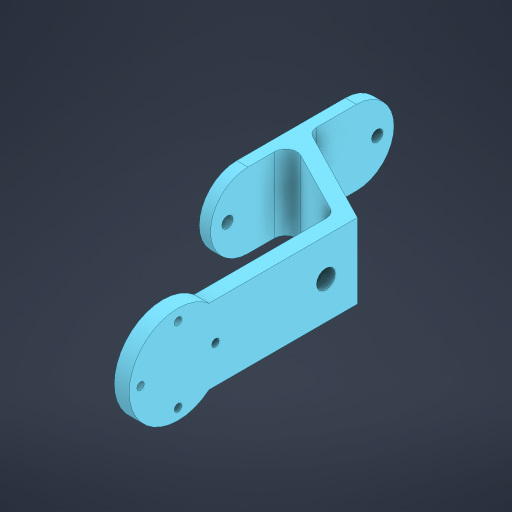
# Autodesk Inventor part: acople_3
Saved by Autodesk Inventor 2023.1 (Build 271208000, 208)
## iProperties
Created: 2022-10-29
Part Number: acople_3
Material: Generic
Document SubType Name: Modeling
Designer: amtat
Density: 1 g/cm^3
Appearance: Default
Author: amtat
Autodesk Inventor part; units mm, degrees
ref_plane "YZ Plane" through (0, 0, 0) normal (1, 0, 0) x (0, 1, 0)
ref_plane "XZ Plane" through (0, 0, 0) normal (0, 1, 0) x (-1, 0, 0)
ref_plane "XY Plane" through (0, 0, 0) normal (0, 0, 1) x (1, 0, 0)
sketch "Sketch1" plane through (0, 0, 0) normal (1, 0, 0) x (0, 1, 0)
  circle A0 centre (0, 0) radius 1.5
  line L0 (0, 0) -> (0, -40)
  circle A1 centre (0, -40) radius 1.5
  line L1 (0, 1.5) -> (0, 4.5)
  line L2 (0, 4.5) -> (0, -5.5)
  arc A2 (10, -5.5) -> (0, -15.5) centre (0, -5.5) ccw
  line L3 (0, -41.5) -> (0, -44.5)
  line L4 (0, -44.5) -> (0, -34.5)
  arc A3 (0, -24.5) -> (10, -34.5) centre (0, -34.5) ccw
  line L5 (0, -34.5) -> (10, -34.5)
  line L6 (0, -5.5) -> (10, -5.5)
  line L7 (10, -5.5) -> (10, -34.5)
  line L8 (-10, -5.5) -> (-10, -34.5)
  dimension "d0" = 3
  dimension "d2" = 3
  dimension "d1" = 40
  dimension "d4" = 3
  dimension "d5" = 10
  dimension "d6" = 3
  dimension "d7" = 10
  constraints: 18 end point, 8 point on circle, 6 point on line, 4 coincident, 2 centre point, 2 vertical, 2 vertical alignment, 1 parallel, 1 perpendicular, 1 tangent, 4 other
  measures "d1" distance of L0.start L0.end
  measures "d4" distance of L1.start L1.end
  measures "d5" distance of L1.end L2.end
  measures "d6" distance of L3.start L3.end
  measures "d7" distance of L3.end L4.end
extrude "Extrusion1" add sketch "Sketch1" along normal blind 3 contours A0 L1 A2 L6 L0 | A0 L0 A2 L1 | L6 L7 L5 L0 | A2 L0 A3 L8 | A3 L3 A1 L0 L5 | A3 L0 A1 L3
sketch "Sketch2" plane through (0, 10, -5.5) normal (0, 1, 0) x (1, 0, 0)
  line L0 (0, 29) -> (0, 0) projected
  line L1 (0, 0) -> (3, 0) projected
  line L2 (3, 29) -> (3, 0) projected
  line L3 (0, 29) -> (3, 29) projected
  line L4 (0, 0) -> (3, 0) projected
  line L5 (0, 0) -> (25.3, 0)
  line L6 (25.3, 0) -> (29.3, 0)
  line L7 (0, -10) -> (3, -10) projected
  line L8 (29.3, 0) -> (29.3, -50)
  line L9 (29.3, -50) -> (25.3, -50)
  line L10 (25.3, -50) -> (25.3, 0)
  point P0 (0, -5.5)
  dimension "d10" = 25.3
  dimension "d11" = 4
  dimension "d12" = 50
  dimension "d13" = 4
  constraints: 10 end point, 2 horizontal, 1 perpendicular, 1 vertical
  measures "d10" distance of L0.end L5.end
  measures "d11" distance of L5.end L6.end
  measures "d12" distance of L6.end L8.end
  measures "d13" distance of L8.end L9.end
extrude "Extrusion2" add sketch "Sketch2" against normal blind 20 contours L6 L8 L9 L10
sketch "Sketch3" plane through (25.3, 10, -5.5) normal (-1, 0, 0) x (0, 0, 1)
  circle A0 centre (5.5, -10) radius 1.5 projected
  circle A1 centre (5.5, -10) radius 1.5 projected
  line L0 (5.5, -10) -> (12, -10)
  line L1 (12, -10) -> (12, 0)
  line L2 (0, 0) -> (50, 0) projected
  line L3 (12, -10) -> (12, -20)
  line L4 (50, -20) -> (0, -20) projected
  line L5 (12, -10) -> (32, -10)
  line L6 (32, -10) -> (45, -10)
  circle A2 centre (45, -10) radius 13
  dimension "d16" = 6.5
  dimension "d17" = 20
  dimension "d18" = 13
  constraints: 10 end point, 3 horizontal, 3 point on line, 1 coincident, 1 horizontal alignment, 1 perpendicular, 2 other
  measures "d16" distance of L0.start L0.end
  measures "d17" distance of L0.end L5.end
  measures "d18" distance of L5.end L6.end
extrude "Extrusion3" add sketch "Sketch3" against normal blind 4 contours A2
sketch "Sketch4" plane through (25.3, -10, -5.5) normal (-1, 0, 0) x (0, 0, 1)
  arc A0 (36.6934, 0) -> (36.6934, 20) centre (45, 10) ccw projected
  line L0 (45, 10) -> (35, 10)
  line L1 (45, 10) -> (45, 20)
  line L2 (45, 10) -> (55, 10)
  line L3 (45, 10) -> (45, 0)
  circle A1 centre (45, 0) radius 0.5
  circle A2 centre (35, 10) radius 0.5
  circle A3 centre (45, 20) radius 0.5
  circle A4 centre (55, 10) radius 0.5
  point P0 (5.5, 10)
  dimension "d21" = 10
  dimension "d22" = 10
  dimension "d23" = 10
  dimension "d24" = 1
  dimension "d25" = 1
  dimension "d26" = 1
  dimension "d27" = 1
  constraints: 8 end point, 4 centre point, 4 coincident, 2 horizontal, 2 vertical
  measures "d21" distance of L0.start L0.end
  measures "d22" distance of L0.start L2.end
  measures "d23" distance of L0.start L3.end
  measures "d24" diameter of A1
  measures "d25" diameter of A2
  measures "d26" diameter of A3
  measures "d27" diameter of A4
extrude "Extrusion4" cut sketch "Sketch4" against normal blind 4
sketch "Sketch6" plane through (0, 10, -5.5) normal (0, 1, 0) x (1, 0, 0)
  line L0 (0, 29) -> (0, 0) projected
  line L1 (0, 0) -> (3, 0) projected
  line L2 (3, 29) -> (3, 0) projected
  line L3 (0, 29) -> (3, 29) projected
  line L4 (25.3, 0) -> (3, 16.5) projected
  line L5 (19.8983, 3.9968) -> (29.3, -2.9596)
  line L6 (29.3, -36.6934) -> (29.3, 0) projected
  point P0 (0, -5.5)
  constraints: 2 end point, 2 point on line
extrude "Extrusion6" [suppressed]
sketch "Sketch7" plane through (29.3, 0, 39.5) normal (1, 0, 0) x (0, 0, -1)
  line L0 (8.3066, 10) -> (45, 10) projected
  arc A0 (8.3066, 10) -> (8.3066, -10) centre (0, 0) ccw projected
  line L1 (45, -10) -> (8.3066, -10) projected
  circle A1 centre (0, -10) radius 0.5 projected
  circle A2 centre (0, 10) radius 0.5 projected
  circle A3 centre (-10, 0) radius 0.5 projected
  circle A4 centre (10, 0) radius 0.5 projected
  circle A5 centre (0, 10) radius 1
  circle A6 centre (10, 0) radius 0.5 projected
  circle A7 centre (10, 0) radius 1
  circle A8 centre (-10, 0) radius 1
  circle A9 centre (0, -10) radius 1
  line L2 (45, 10) -> (45, -10) projected
  point P0 (39.5, 0)
  dimension "d40" = 2
  dimension "d41" = 2
  dimension "d42" = 2
  dimension "d43" = 2
  constraints: 4 centre point, 4 coincident
  measures "d40" diameter of A5
  measures "d41" diameter of A7
  measures "d42" diameter of A8
  measures "d43" diameter of A9
extrude "Extrusion7" cut sketch "Sketch7" against normal blind 10 contours A3 | A4 | A5 | A7 | A8 | A9
sketch "Sketch8" plane through (29.3, 10, -5.5) normal (0, 0, -1) x (-1, 0, 0)
  line L0 (0, 0) -> (4, 0) projected
  line L1 (0, 0) -> (0, -20) projected
  line L2 (4, -20) -> (0, -20) projected
  line L3 (4, 0) -> (4, -20) projected
  point P0 (29.3, -10)
extrude "Extrusion8" add sketch "Sketch8" along normal blind 5
sketch "Sketch9" plane through (0, 10, -5.5) normal (0, 1, 0) x (1, 0, 0)
  line L0 (0, 29) -> (0, 0) projected
  line L1 (0, 0) -> (3, 0) projected
  line L2 (3, 29) -> (3, 0) projected
  line L3 (0, 29) -> (3, 29) projected
  line L4 (3, 0) -> (3, 29) projected
  line L5 (3, 0) -> (3, 14.5)
  line L6 (25.3, -36.6934) -> (29.3, -36.6934) projected
  line L7 (29.3, -36.6934) -> (29.3, 5) projected
  line L8 (25.3, 5) -> (29.3, 5) projected
  line L9 (25.3, 5) -> (25.3, -36.6934) projected
  line L10 (3, 14.5) -> (3, 16.5)
  line L11 (25.3, -36.6934) -> (25.3, 5) projected
  line L12 (3, 16.5) -> (25.3, 5)
  line L13 (18.1684, 8.6777) -> (16.3351, 5.1226)
  line L14 (8.3049, 13.7643) -> (6.4715, 10.2092)
  line L15 (16.3351, 5.1226) -> (3, 11.9994)
  line L16 (6.4715, 10.2092) -> (25.3, 0.4994)
  point P0 (0, -5.5)
  point P1 (3, 11.9994)
  point P2 (16.3351, 5.1226)
  point P3 (25.3, 0.4994)
  dimension "d48" = 14.5
  dimension "d49" = 2
  dimension "d51" = 4
  dimension "d52" = 4
  constraints: 14 end point, 6 point on line, 2 perpendicular, 1 midpoint
  measures "d48" distance of L1.end L5.end
  measures "d49" distance of L5.end L10.end
  measures "d51" distance of L13.start L13.end
  measures "d52" distance of L14.start L14.end
extrude "Extrusion9" add sketch "Sketch9" against normal blind 20 contours L12 L14 L15 L2 | L12 L13 L15 L14 | L12 L9 L16 L13
sketch "Sketch10" plane through (0, 10, -5.5) normal (0, 1, 0) x (1, 0, 0)
  line L0 (0, 29) -> (0, 0) projected
  line L1 (0, 0) -> (3, 0) projected
  line L2 (3, 11.9994) -> (3, 0) projected
  line L3 (3, 11.9994) -> (25.3, 0.4994) projected
  line L4 (25.3, 0.4994) -> (25.3, -36.6934) projected
  line L5 (25.3, -36.6934) -> (29.3, -36.6934) projected
  line L6 (29.3, -36.6934) -> (29.3, 5) projected
  line L7 (25.3, 5) -> (29.3, 5) projected
  line L8 (25.3, 5) -> (3, 16.5) projected
  line L9 (3, 29) -> (3, 16.5) projected
  line L10 (0, 29) -> (3, 29) projected
  line L11 (3, 16.5) -> (25.3, 5) projected
  line L12 (3, 16.5) -> (29.3, 2.9372)
  line L13 (29.3, -36.6934) -> (29.3, 5) projected
  point P0 (0, -5.5)
  point P1 (29.3, 2.9372)
  constraints: 2 end point, 1 point on line
extrude "Extrusion10" cut sketch "Sketch10" against normal blind 20 contours L7 L6 L12
sketch "Sketch11" plane through (29.3, 0, 39.5) normal (1, 0, 0) x (0, 0, -1)
  circle A0 centre (39.5, 0) radius 1.5 projected
  circle A1 centre (39.5, 0) radius 2.5
  dimension "d57" = 5
  constraints: 1 centre point, 1 coincident
  measures "d57" diameter of A1
extrude "Extrusion11" cut sketch "Sketch11" against normal blind 5 contours A0 | A1
fillet "Fillet3" radius 3 3 edges at (3, 0, -17.4994) (3, 0, -22) (25.3, 0, -5.9994)
body "Solid1"
